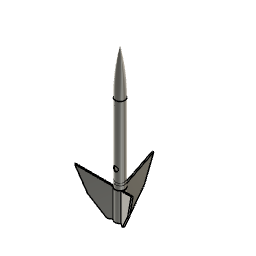
xb auk 12 (Autodesk Fusion 360 design; units mm, degrees)
Autodesk Fusion 360 part; units mm, degrees
sketch "Sketch1" plane through (0, 0, 0) normal (0, 0, 1) x (1, 0, 0)
  circle A0 centre (0, 0) radius 9
  circle A1 centre (0, 0) radius 10.5
  line L0 (1.5, 70) -> (-1.5, 70)
  line L1 (1.5, 70) -> (-1.5, -70) construction
  line L2 (-1.5, 70) -> (1.5, -70) construction
  line L3 (-1.5, 0) -> (1.5, 0)
  line L4 (1.5, 0) -> (1.5, 70)
  line L5 (-1.5, 70) -> (-1.5, 0)
  line L6 (-59.8718, -36.299) -> (0.75, -1.299)
  line L7 (-61.3718, -33.701) -> (-59.8718, -36.299)
  line L8 (-0.75, 1.299) -> (-61.3718, -33.701)
  line L9 (61.3718, -33.701) -> (0.75, 1.299)
  line L10 (59.8718, -36.299) -> (61.3718, -33.701)
  line L11 (-0.75, -1.299) -> (59.8718, -36.299)
  dimension "d1" = 18
  dimension "d2" = 21
  dimension "d3" = 3
  dimension "d4" = 140
  dimension "d6" = 360
  constraint coincident A0.centre A1.centre
  constraint concentric A0 A1
  constraint horizontal L0
  constraint perpendicular L0 L5
  constraint coincident L1 A0.centre
  constraint coincident L2 A0.centre
  measures "d1" diameter of A0
  measures "d2" diameter of A1
  measures "d3" distance of L1.end L2.end
  measures "d4" distance of L0.end L1.end
extrude "Extrude1" add sketch "Sketch1" along normal blind 70 contours A0 A1 L4 L9 | A0 A1 L4 L5 | A0 A1 L9 L11 | A0 A1 L5 L8 | A0 A1 L6 L11 | A0 A1 L6 L8 makes body 1
extrude "Extrude2" add sketch "Sketch1" along normal blind 90 contours A1 L0 L4 L5 | A1 L9 L10 L11 | A1 L6 L7 L8 bodies 1
sketch "Sketch2" plane through (0, 0, 70) normal (0, 0, 1) x (-1, 0, 0)
  circle A0 centre (0, 0) radius 9
  arc A1 (-9.75, 3.8971) -> (-1.5, -10.3923) centre (0, 0) ccw
  arc A2 (-1.5, -10.3923) -> (1.5, -10.3923) centre (0, 0) ccw
  arc A3 (1.5, -10.3923) -> (9.75, 3.8971) centre (0, 0) ccw
  arc A4 (9.75, 3.8971) -> (8.25, 6.4952) centre (0, 0) ccw
  arc A5 (8.25, 6.4952) -> (-8.25, 6.4952) centre (0, 0) ccw
  arc A6 (-8.25, 6.4952) -> (-9.75, 3.8971) centre (0, 0) ccw
  circle A7 centre (0, 0) radius 8
  circle A8 centre (0, 0) radius 10.5
  constraint concentric A0 A7
  constraint concentric A7 A8
sketch "Sketch3" plane through (0, 0, 70) normal (0, 0, 1) x (1, 0, 0)
extrude "Extrude3" add sketch "Sketch2" along normal blind 4 contours A0 | A1 A2 A3 A4 A5 A6 A8 bodies 1
sketch "Sketch4" plane through (0, 0, 74) normal (0, 0, 1) x (-1, 0, 0)
  circle A0 centre (0, 0) radius 8
  arc A1 (-1.5, -10.3923) -> (1.5, -10.3923) centre (0, 0) ccw
  arc A2 (1.5, -10.3923) -> (9.75, 3.8971) centre (0, 0) ccw
  arc A3 (9.75, 3.8971) -> (8.25, 6.4952) centre (0, 0) ccw
  arc A4 (8.25, 6.4952) -> (-8.25, 6.4952) centre (0, 0) ccw
  arc A5 (-8.25, 6.4952) -> (-9.75, 3.8971) centre (0, 0) ccw
  arc A6 (-9.75, 3.8971) -> (-1.5, -10.3923) centre (0, 0) ccw
  circle A7 centre (0, 0) radius 9
  constraint coincident A0.centre A1.centre
sketch "Sketch5" plane through (0, 0, 0) normal (0, 1, 0) x (1, 0, 0)
sketch "Sketch6" plane through (0, 0, 0) normal (1, 0, 0) x (0, 1, 0)
  line L0 (20, 0) -> (50, 40)
  line L1 (50, 40) -> (70, 90)
  line L2 (70, 90) -> (100, 90)
  line L3 (100, 90) -> (100, -10)
  line L4 (100, -10) -> (20, -10)
  line L5 (20, -10) -> (20, 0)
  constraint horizontal L2
  constraint perpendicular L2 L3
  constraint perpendicular L3 L4
  constraint perpendicular L4 L5
revolve "Revolve1" cut sketch "Sketch6" angle 360 about axis through (0, 0, 1.75) along (0, 0, 1) bodies 1
sketch "Sketch7" plane through (0, 0, 0) normal (1, 0, 0) x (0, 1, 0)
  line L0 (10, 60) -> (70, 90)
  line L1 (70, 90) -> (70, 120)
  line L2 (70, 120) -> (10, 120)
  line L3 (10, 120) -> (10, 60)
  constraint vertical L1
  constraint perpendicular L1 L2
  constraint perpendicular L2 L3
revolve "Revolve2" cut sketch "Sketch7" angle 360 about axis through (0, 0, 1.75) along (0, 0, 1) bodies 1
sketch "Sketch8" plane through (0, 0, 74) normal (0, 0, 1) x (-1, 0, 0)
  circle A0 centre (0, 0) radius 10
  circle A1 centre (0, 0) radius 8
  circle A2 centre (0, 0) radius 10
  circle A3 centre (0, 0) radius 9
  constraint coincident A0.centre A1.centre
  constraint concentric A2 A3
extrude "Extrude5" add sketch "Sketch8" along normal blind 150 contours A0 A2 bodies 1
sketch "Sketch9" plane through (0, 0, 0) normal (1, 0, 0) x (0, 1, 0)
  line L0 (10, 224) -> (8, 224)
  line L1 (8, 224) -> (8, 212)
  line L2 (8, 212) -> (-8, 212)
  line L3 (-8, 212) -> (-8, 224)
  line L4 (-8, 224) -> (-10, 224)
  line L5 (0, 212) -> (0, 320)
  arc A0 (10, 224) -> (0, 320) centre (-394.6442, 230.3704) ccw
  arc A1 (0, 320) -> (-10, 224) centre (394.6442, 230.3704) ccw
  constraint horizontal L0
  constraint perpendicular L0 L1
  constraint perpendicular L1 L2
  constraint perpendicular L2 L3
  constraint perpendicular L3 L4
  constraint midpoint L2 L5.start
  constraint perpendicular L2 L5
  constraint symmetric L0.start L5 L4.end
  constraint symmetric A0.end L5 A1.start
  constraint symmetric L5 A0 A1
revolve "Revolve3" add sketch "Sketch9" angle 360 about axis through (0, 0, 212) along (0, 0, 1) separate body contours L0 L1 L2 L5 A0 makes body 2
sketch "Sketch10" plane through (0, 0, 0) normal (1, 0, 0) x (0, 1, 0)
sketch "Sketch11" plane through (0, 0, 0) normal (0, 0, 1) x (1, 0, 0)
  circle A0 centre (0, 0) radius 10.5
  circle A1 centre (-11.4411, 6.1727) radius 2.5
  line L0 (-9.707, 9.2129) -> (-7.1066, 7.7296)
  line L1 (-11.4411, 6.1727) -> (-9.707, 9.2129)
  line L2 (-11.4411, 6.1727) -> (-12.5851, 6.8252) construction
  line L3 (-11.4411, 6.1727) -> (-13.1752, 3.1325)
  line L4 (-13.1752, 3.1325) -> (-10.3862, 1.5416)
  arc A2 (-9.707, 9.2129) -> (-13.1752, 3.1325) centre (-11.4411, 6.1727) ccw
  arc A3 (-10.0773, 2.9493) -> (-7.9983, 6.8028) centre (-11.4411, 6.1727) ccw
  dimension "d20" = 5
  constraint tangent A0 A1
  constraint coincident A0 L0.end
  constraint tangent L0 A2
  constraint coincident A1.centre L1.start
  constraint perpendicular L1 L2
  constraint parallel L1 L3
  constraint coincident A0 L4.end
  constraint tangent L4 A2
  constraint concentric A1 A2
  constraint coincident A0 A3.end
  constraint coincident A0 A3.start
  constraint concentric A2 A3
  measures "d20" diameter of A1
extrude "Extrude6" add sketch "Sketch11" along normal blind 50 contours A0 A1 L0 L1 | A0 A1 L3 L4 | A1 L1 L3 A2 bodies 1
ref_plane "WorkPlane1" through (0, -10, 98.3205) normal (0, -1, 0) x (1, 0, 0)
sketch "Sketch12" plane through (0, -10, 98.3205) normal (0, -1, 0) x (1, 0, 0)
  circle A0 centre (0, 0) radius 5
  dimension "d25" = 10
  constraint coincident A0.centre origin
  measures "d25" diameter of A0
extrude "Extrude7" cut sketch "Sketch12" against normal blind 10 bodies 1
sketch "Sketch13" plane through (0, 0, 212) normal (0, 0, -1) x (1, 0, 0)
  circle A0 centre (0, 0) radius 8
  circle A1 centre (-5, 0) radius 1.5
  line L0 (-8, 0) -> (-8, 5)
  dimension "d28" = 3
  constraint coincident A0 L0.start
  constraint tangent A0 L0
  constraint vertical L0
  measures "d28" diameter of A1
revolve "Revolve4" cut sketch "Sketch13" angle 360 about axis through (-8, 0, 212) along (0, -1, 0) contours A1 bodies 2
chamfer "Chamfer1" distance 1 angle 45 1 edges at (-8.3909, 3.2545, 70) on bodies 1
